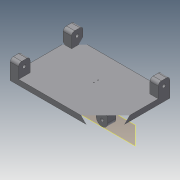
# Autodesk Inventor part: Part4
Saved by Autodesk Inventor 2014 SP1 (Build 180222100, 222)
## iProperties
Created: 2014-03-25
Part Number: Part4
Material: Generic
Document SubType Name: Modeling
Designer: tom
Density: 1 g/cm^3
Appearance: Default
Author: tom
Autodesk Inventor part; units mm, degrees
ref_plane "YZ Plane" through (0, 0, 0) normal (1, 0, 0) x (0, 1, 0)
ref_plane "XZ Plane" through (0, 0, 0) normal (0, 1, 0) x (-1, 0, 0)
ref_plane "XY Plane" through (0, 0, 0) normal (0, 0, 1) x (1, 0, 0)
ref_plane "Work Plane1" through (-106.5416, 98.4713, 124.9427) normal (0, 0, 1) x (1, 0, 0)
sketch "Sketch1" plane through (-106.5416, 98.4713, 124.9427) normal (0, 0, 1) x (1, 0, 0)
  circle A0 centre (19.5, 13) radius 1.5 projected
  arc A1 (52.5, 10.25) -> (37.5, 10.25) centre (45, 10.25) ccw projected
  circle A2 centre (19.5, 13) radius 5.5 construction
  line L0 (45, 10.25) -> (45, 17.75) construction
  line L1 (45, 17.75) -> (45, 23.75) construction
  line L2 (45, 23.75) -> (19.5, 23.75) construction
  arc A3 (14.0371, 13.6378) -> (25, 13) centre (19.5, 13) ccw
  line L3 (25, 13) -> (25, 23.75)
  circle A4 centre (19.5, 13) radius 1.5
  line L4 (14.0028, 12.8238) -> (14.0028, 23.75)
  line L5 (14.0028, 23.75) -> (25, 23.75)
  point P0 (106.5416, -98.4713)
  point P1 (14.0469, 12.2829)
  dimension "d0" = 11
  dimension "d4" = 10.75
  constraints: 12 end point, 8 point on circle, 3 centre point, 3 coincident, 2 collinear, 2 concentric, 2 perpendicular, 2 tangent, 1 parallel, 1 point on line
  measures "d0" diameter of A2
  measures "d4" distance from line of L5 A0.centre
extrude "Extrusion1" add sketch "Sketch1" along normal blind 8
pattern_linear "Rectangular Pattern2" count 2 spacing 51 along (1, 0, 0) count 2 spacing 20 along (0, 0, -1) of "Extrusion1"
sketch "Sketch3" plane through (-92.5388, 122.2213, 124.9427) normal (0, 1, 0) x (1, 0, 0)
  line L0 (0, 20) -> (61.9972, 20) construction
  line L1 (0, 20) -> (0, -8) construction
  line L2 (0, 6) -> (86.2224, 6) construction
  line L3 (31, 37) -> (31, -25) construction
  line L4 (31, -25) -> (-14.75, -25) construction
  line L5 (31, -25) -> (76.75, -25) construction
  line L6 (76.75, -25) -> (76.75, 37)
  line L7 (76.75, 37) -> (-14.75, 37)
  line L8 (-14.75, 37) -> (-14.75, -25)
  line L9 (-14.75, -25) -> (76.75, -25)
  point P0 (92.5388, 124.9427)
  dimension "d29" = 45.75
  dimension "d30" = 45.75
  dimension "d31" = 62
  constraints: 20 end point, 5 perpendicular, 2 equal length, 1 midpoint
  measures "d29" distance of L3.end L4.end
  measures "d30" distance of L3.end L5.end
  measures "d31" distance of L5.end L6.end
extrude "Extrusion3" add sketch "Sketch3" against normal blind 5
ref_plane "Work Plane2" through (-60.8166, 113.6367, 119.7132) normal (0, 0.9135, -0.4067) x (-1, 0, 0)
sketch "Sketch4" plane through (-60.8166, 113.6367, 119.7132) normal (0, 0.9135, -0.4067) x (-1, 0, 0)
  circle A0 centre (-0.457, 0.457) radius 0.457 projected
  circle A1 centre (-0.457, 0.457) radius 0.457
  circle A2 centre (-0.457, 0.457) radius 0.375
  point P0 (-60.8166, -155.5837)
  dimension "d32" = 0.75
  constraints: 2 centre point, 2 coincident, 1 concentric
  measures "d32" diameter of A2
extrude "Extrusion4" cut sketch "Sketch4" along normal blind 15 contours A2
pattern_linear "Rectangular Pattern3" count 2 spacing 4 along (0, 0, -1) of "Extrusion4"
sketch "Sketch5" plane through (-107.2888, 122.2213, 149.9427) normal (0, 1, 0) x (1, 0, 0)
  line L0 (0, 0) -> (0, 62) projected
  line L1 (0, 62) -> (91.5, 62) projected
  line L2 (0, 62) -> (0, 51)
  line L3 (0, 51) -> (8, 51)
  line L4 (8, 51) -> (8, 62)
  line L5 (0, 62) -> (8, 62)
  point P0 (107.2888, 149.9427)
  dimension "d38" = 11
  dimension "d39" = 8
  constraints: 8 end point, 3 perpendicular, 2 point on line
  measures "d38" distance of L0.end L2.end
  measures "d39" distance of L2.end L3.end
extrude "Extrusion5" add sketch "Sketch5" along normal blind 13.5
sketch "Sketch6" plane through (-99.2888, 122.2213, 98.9427) normal (1, 0, 0) x (0, 0, -1)
  line L0 (11, 0) -> (11, 13.5) projected
  line L1 (0, 13.5) -> (11, 13.5) projected
  circle A0 centre (5.5, 8) radius 1.5
  dimension "d42" = 3
  dimension "d43" = 5.5
  dimension "d44" = 5.5
  constraints: 1 centre point
  measures "d42" diameter of A0
  measures "d43" distance from line of L1 A0.centre
  measures "d44" distance from line of L0 A0.centre
extrude "Extrusion6" cut sketch "Sketch6" against normal blind 24.6
fillet "Fillet1" radius 3 2 edges at (-103.2888, 135.7213, 98.9427) (-103.2888, 135.7213, 87.9427)
pattern_linear "Rectangular Pattern4" count 2 spacing 51 along (0, 0, 1) count 2 spacing 83.5 along (1, 0, 0) of "Extrusion5", "Fillet1", "Extrusion6"
body "Solid1"
